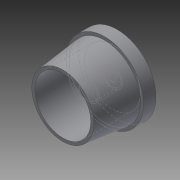
# Autodesk Inventor part: pot
Saved by Autodesk Inventor 2014 (Build 180170000, 170)
## iProperties
Created: 2014-04-02
Part Number: pot
Material: Generic
Document SubType Name: Modeling
Designer: jferner
Density: 1 g/cm^3
Appearance: Default
potOpeningDia: 36.000 mm
Author: jferner
Autodesk Inventor part; units mm, degrees
ref_plane "YZ Plane" through (0, 0, 0) normal (1, 0, 0) x (0, 1, 0)
ref_plane "XZ Plane" through (0, 0, 0) normal (0, 1, 0) x (-1, 0, 0)
ref_plane "XY Plane" through (0, 0, 0) normal (0, 0, 1) x (1, 0, 0)
sketch "Sketch2" plane through (0, 0, 0) normal (0, 0, 1) x (1, 0, 0)
  line L0 (0, 0) -> (0, 35)
  line L1 (0, 35) -> (25, 35)
  line L2 (25, 35) -> (25, 27)
  line L3 (25, 27) -> (23, 27)
  line L4 (23, 27) -> (20, 0)
  line L5 (20, 0) -> (0, 0)
  dimension "d1" = 20
  dimension "d2" = 25
  dimension "d3" = 2
  dimension "d4" = 8
  dimension "d5" = 35
  constraints: 12 end point, 3 parallel, 1 perpendicular, 1 vertical
  measures "d1" distance of L4.end L0.start
  measures "d2" distance of L0.end L1.end
  measures "d3" distance of L2.end L3.end
  measures "d4" distance of L1.end L2.end
  measures "d5" distance of L0.start L0.end
revolve "Revolution1" add sketch "Sketch2" angle 360 about axis through (0, 0, 0) along (0, 1, 0)
sketch "Sketch3" plane through (0, 35, 0) normal (0, 1, 0) x (1, 0, 0)
  circle A0 centre (0, 0) radius 25 projected
  circle A1 centre (0, 0) radius 1
  dimension "d7" = 2
  constraints: 1 centre point, 1 coincident
  measures "d7" diameter of A1
extrude "Extrusion1" cut sketch "Sketch3" against normal through all contours A1
sketch "Sketch4" plane through (0, 0, 0) normal (0, -1, 0) x (1, 0, 0)
  circle A0 centre (0, 0) radius 1 projected
  circle A1 centre (0, 0) radius 20 projected
  circle A2 centre (0, 0) radius 18
  dimension "d10" = 2
  dimension "potOpeningDia" = 36
  constraints: 1 centre point, 1 coincident
  measures "d10" radial gap between concentric circles of A1 A2
  measures "potOpeningDia" diameter of A2
extrude "Extrusion2" cut sketch "Sketch4" against normal blind 32 contours A2
sketch "Sketch5" plane through (0, 32, 0) normal (0, -1, 0) x (1, 0, 0)
  circle A0 centre (0, 0) radius 1 projected
  circle A1 centre (0, 0) radius 18 projected
  circle A2 centre (0, 0) radius 2.5
  dimension "d13" = 5
  constraints: 1 centre point, 1 coincident
  measures "d13" diameter of A2
extrude "Extrusion3" add sketch "Sketch5" along normal blind 5 contours A2
sketch "Sketch6" plane through (0, 32, 0) normal (0, -1, 0) x (1, 0, 0)
  circle A0 centre (0, 0) radius 18 projected
  circle A1 centre (0, 0) radius 5.5
  circle A2 centre (0, 0) radius 6.5
  dimension "d17" = 11
  dimension "d18" = 1
  constraints: 2 centre point, 2 coincident
  measures "d17" diameter of A1
  measures "d18" radial gap between concentric circles of A2 A1
extrude "Extrusion4" add sketch "Sketch6" along normal blind 15 contours A2
body "Solid1"
